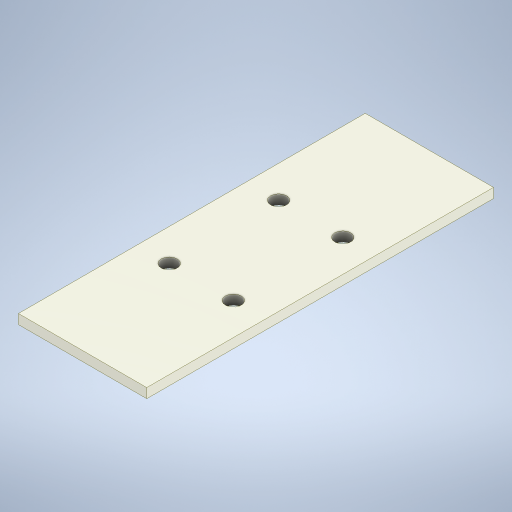
# Autodesk Inventor part: slider_puffer.iam
Saved by Autodesk Inventor 2024 (Build 280153000, 153)
## iProperties
Created: 2025-12-26
Part Number: slider_puffer.iam
Material: Polytetrafluoroethylene
Document SubType Name: Modeling
Designer: schar
Density: 2.02 g/cm^3
Appearance: Smooth - Ivory
Author: schar
Autodesk Inventor part; units mm, degrees
ref_plane "YZ Plane" through (0, 0, 0) normal (1, 0, 0) x (0, 1, 0)
ref_plane "XZ Plane" through (0, 0, 0) normal (0, 1, 0) x (-1, 0, 0)
ref_plane "XY Plane" through (0, 0, 0) normal (0, 0, 1) x (1, 0, 0)
sketch "Sketch1" plane through (0, 0, 0) normal (0, 1, 0) x (-1, 0, 0)
  line L0 (20, 34.056) -> (-20, 34.056)
  line L1 (-20, 34.056) -> (-20, -34.056)
  line L2 (-20, -34.056) -> (20, -34.056)
  line L3 (20, -34.056) -> (20, 34.056)
  line L4 (20, 34.056) -> (-20, -34.056) construction
  line L5 (-20, 34.056) -> (20, -34.056) construction
  line L6 (-20, 34.056) -> (-10, 34.056)
  line L7 (-10, 34.056) -> (-10, 17.056)
  line L8 (-10, 17.056) -> (-20, 17.056)
  line L9 (-20, 17.056) -> (-20, 34.056)
  line L10 (20, 34.056) -> (10, 34.056)
  line L11 (10, 34.056) -> (10, 17.056)
  line L12 (10, 17.056) -> (20, 17.056)
  line L13 (20, 17.056) -> (20, 34.056)
  line L14 (20, -34.056) -> (10, -34.056)
  line L15 (10, -34.056) -> (10, -17.056)
  line L16 (10, -17.056) -> (20, -17.056)
  line L17 (20, -17.056) -> (20, -34.056)
  line L18 (-20, -34.056) -> (-10, -34.056)
  line L19 (-10, -34.056) -> (-10, -17.056)
  line L20 (-10, -17.056) -> (-20, -17.056)
  line L21 (-20, -17.056) -> (-20, -34.056)
  circle A0 centre (-10, 17.056) radius 2.5
  circle A1 centre (10, 17.056) radius 2.5
  circle A2 centre (10, -17.056) radius 2.5
  circle A3 centre (-10, -17.056) radius 2.5
  line L22 (20, 34.056) -> (-20, 34.056)
  line L23 (-20, 34.056) -> (-20, 54.056)
  line L24 (-20, 54.056) -> (20, 54.056)
  line L25 (20, 54.056) -> (20, 34.056)
  line L26 (20, -34.056) -> (-20, -34.056)
  line L27 (-20, -34.056) -> (-20, -54.056)
  line L28 (-20, -54.056) -> (20, -54.056)
  line L29 (20, -54.056) -> (20, -34.056)
  point P0 (0, 0)
  dimension "d0" = 40
  dimension "d1" = 68.112
  dimension "d2" = 10
  dimension "d3" = 17
  dimension "d4" = 10
  dimension "d5" = 17
  dimension "d6" = 10
  dimension "d7" = 17
  dimension "d8" = 10
  dimension "d9" = 17
  dimension "d10" = 5
  dimension "d11" = 5
  dimension "d12" = 5
  dimension "d13" = 5
  dimension "d14" = 20
  dimension "d15" = 20
  constraints: 60 end point, 14 parallel, 7 horizontal, 7 perpendicular, 4 centre point, 4 coincident, 2 midpoint, 1 point on line
  measures "d0" distance of L2.end L1.end
  measures "d1" distance of L1.end L0.end
  measures "d2" distance of L7.end L8.end
  measures "d3" distance of L6.end L7.end
  measures "d4" distance of L12.end L11.end
  measures "d5" distance of L11.end L10.end
  measures "d6" distance of L15.end L16.end
  measures "d7" distance of L14.end L15.end
  measures "d8" distance of L20.end L19.end
  measures "d9" distance of L19.end L18.end
  measures "d10" diameter of A0
  measures "d11" diameter of A1
  measures "d12" diameter of A2
  measures "d13" diameter of A3
  measures "d14" distance of L22.end L23.end
  measures "d15" distance of L27.end L26.end
extrude "Extrusion1" add sketch "Sketch1" along normal blind 3 contours L3 L12 A1 L11 L0 | L0 L23 L24 L25 | L11 A1 L12 L3 L16 A2 L15 L2 L19 A3 L20 L1 L8 A0 L7 L0 | L7 A0 L8 L1 L0 | L3 L2 L15 A2 L16 | L29 L28 L27 L2 | L20 A3 L19 L2 L1
body "Solid1"
